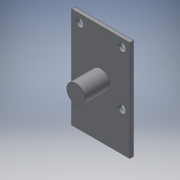
# Autodesk Inventor part: joystick
Saved by Autodesk Inventor 2019 (Build 230136000, 136)
## iProperties
Created: 2021-03-13
Part Number: joystick
Material: Generic
Document SubType Name: Modeling
Designer: Vijay
Density: 1 g/cm^3
Appearance: Default
Author: Vijay
Autodesk Inventor part; units mm, degrees
ref_plane "YZ Plane" through (0, 0, 0) normal (1, 0, 0) x (0, 1, 0)
ref_plane "XZ Plane" through (0, 0, 0) normal (0, 1, 0) x (-1, 0, 0)
ref_plane "XY Plane" through (0, 0, 0) normal (0, 0, 1) x (1, 0, 0)
sketch "Sketch1" plane through (0, 0, 0) normal (0, 0, 1) x (1, 0, 0)
  line L0 (149.3695, 15.7093) -> (174.8695, 15.7093)
  line L1 (174.8695, 15.7093) -> (174.8695, -28.3907)
  line L2 (174.8695, -28.3907) -> (149.3695, -28.3907)
  line L3 (149.3695, -28.3907) -> (149.3695, 15.7093)
  circle A0 centre (152.8695, 12.2093) radius 1.75
  circle A1 centre (171.3695, 12.2093) radius 1.75
  circle A2 centre (152.8695, -11.2907) radius 1.75
  circle A3 centre (171.3695, -11.2907) radius 1.75
  line L4 (162.1195, 21.9473) -> (162.1195, -33.4191) construction
  line L5 (144.2972, -9.7907) -> (180.3541, -9.7907) construction
  line L6 (143.6152, 0.7093) -> (182.6159, 0.7093) construction
  line L7 (156.6972, 0.7093) -> (167.6534, 0.7093) construction
  line L8 (167.6534, 0.7093) -> (167.6534, -9.7907) construction
  line L9 (167.6534, -9.7907) -> (156.6972, -9.7907) construction
  line L10 (156.6972, -9.7907) -> (156.6972, 0.7093) construction
  line L11 (156.6972, -4.5407) -> (167.6534, -4.5407) construction
  circle A4 centre (162.1753, -4.5407) radius 4
  point P0 (0, 0)
  dimension "d0" = 44.1
  dimension "d1" = 25.5
  dimension "d2" = 3.5
  dimension "d3" = 3.5
  dimension "d4" = 3.5
  dimension "d5" = 3.5
  dimension "d6" = 3.5
  dimension "d7" = 3.5
  dimension "d8" = 3.5
  dimension "d9" = 3.5
  dimension "d10" = 27
  dimension "d11" = 27
  dimension "d12" = 25.5
  dimension "d13" = 10.5
  dimension "d14" = 8
  constraints: 24 end point, 5 centre point, 4 horizontal, 4 parallel, 3 midpoint, 2 perpendicular, 2 point on line, 1 vertical
  measures "d0" distance of L2.end L0.start
  measures "d1" distance of L0.start L0.end
  measures "d2" distance from line of L3 A0.centre
  measures "d3" distance from line of A0.centre L0
  measures "d4" diameter of A0
  measures "d5" diameter of A1
  measures "d6" distance from line of L0 A1.centre
  measures "d7" distance from line of A1.centre L1
  measures "d8" diameter of A2
  measures "d9" diameter of A3
  measures "d10" distance from line of A2.centre L0
  measures "d11" distance from line of A3.centre L0
  measures "d12" distance between parallel lines of L5 L0
  measures "d13" distance between parallel lines of L5 L6
  measures "d14" diameter of A4
extrude "Extrusion1" add sketch "Sketch1" along normal blind 1.6
sketch "Sketch2" plane through (0, 0, 1.6) normal (0, 0, 1) x (1, 0, 0)
  circle A0 centre (162.1753, -4.5407) radius 4 projected
  point P0 (0, 0)
extrude "Extrusion2" add sketch "Sketch2" along normal blind 11
body "Solid1"
